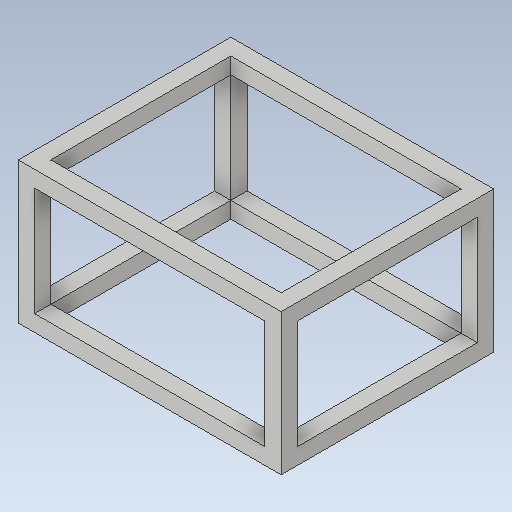
# Autodesk Inventor part: Turning motor housing
Saved by Autodesk Inventor 2020 (Build 240168000, 168)
## iProperties
Created: 2020-10-15
Part Number: Turning motor housing
Material: Generic
Document SubType Name: Modeling
Designer: nabee
Density: 1 g/cm^3
Appearance: Default
Author: nabee
Autodesk Inventor part; units mm, degrees
ref_plane "YZ Plane" through (0, 0, 0) normal (1, 0, 0) x (0, 1, 0)
ref_plane "XZ Plane" through (0, 0, 0) normal (0, 1, 0) x (-1, 0, 0)
ref_plane "XY Plane" through (0, 0, 0) normal (0, 0, 1) x (1, 0, 0)
sketch "Sketch1" plane through (0, 0, 0) normal (0, 0, 1) x (1, 0, 0)
  line L0 (0, 0) -> (322.448, 0)
  line L1 (322.448, 0) -> (322.448, 173.35)
  line L2 (322.448, 173.35) -> (0, 173.35)
  line L3 (0, 173.35) -> (0, 0)
  dimension "d0" = 322.448
  dimension "d1" = 173.35
  constraints: 8 end point, 2 parallel, 1 horizontal, 1 perpendicular
  measures "d0" distance of L2.end L1.end
  measures "d1" distance of L2.end L0.start
extrude "Extrusion1" add sketch "Sketch1" along normal blind 260.725
sketch "Sketch2" plane through (0, 0, 260.725) normal (0, 0, 1) x (1, 0, 0)
  line L0 (20, 153.35) -> (302.448, 153.35)
  line L1 (302.448, 153.35) -> (302.448, 20)
  line L2 (302.448, 20) -> (20, 20)
  line L3 (20, 20) -> (20, 153.35)
  line L4 (322.448, 173.35) -> (0, 173.35) projected
  line L5 (0, 173.35) -> (0, 0) projected
  line L6 (0, 0) -> (322.448, 0) projected
  line L7 (322.448, 0) -> (322.448, 173.35) projected
  dimension "d4" = 20
  dimension "d5" = 20
  dimension "d6" = 20
  dimension "d7" = 20
  constraints: 8 end point, 2 parallel, 1 horizontal, 1 perpendicular
  measures "d4" distance between parallel lines of L4 L0
  measures "d5" distance between parallel lines of L5 L3
  measures "d6" distance between parallel lines of L6 L2
  measures "d7" distance between parallel lines of L7 L1
extrude "Extrusion2" cut sketch "Sketch2" against normal blind 900 contours L0 L1 L2 L3
sketch "Sketch3" plane through (322.448, 0, 0) normal (1, 0, 0) x (0, 0, -1)
  line L0 (-240.725, 153.35) -> (-20, 153.35)
  line L1 (-20, 153.35) -> (-20, 20)
  line L2 (-20, 20) -> (-240.725, 20)
  line L3 (-240.725, 20) -> (-240.725, 153.35)
  line L4 (0, 173.35) -> (-260.725, 173.35) projected
  line L5 (-260.725, 0) -> (-260.725, 173.35) projected
  line L6 (0, 0) -> (-260.725, 0) projected
  line L7 (0, 0) -> (0, 173.35) projected
  dimension "d10" = 20
  dimension "d11" = 20
  dimension "d12" = 20
  dimension "d13" = 20
  constraints: 8 end point, 2 parallel, 1 horizontal, 1 perpendicular
  measures "d10" distance between parallel lines of L4 L0
  measures "d11" distance between parallel lines of L5 L3
  measures "d12" distance between parallel lines of L6 L2
  measures "d13" distance between parallel lines of L7 L1
extrude "Extrusion3" cut sketch "Sketch3" against normal blind 900 contours L0 L1 L2 L3
sketch "Sketch4" plane through (0, 173.35, 0) normal (0, 1, 0) x (1, 0, 0)
  line L0 (20, -20) -> (302.448, -20)
  line L1 (302.448, -20) -> (302.448, -240.725)
  line L2 (302.448, -240.725) -> (20, -240.725)
  line L3 (20, -240.725) -> (20, -20)
  line L4 (322.448, 0) -> (0, 0) projected
  line L5 (0, 0) -> (0, -260.725) projected
  line L6 (322.448, 0) -> (322.448, -260.725) projected
  line L7 (322.448, -260.725) -> (0, -260.725) projected
  dimension "d16" = 20
  dimension "d17" = 20
  dimension "d18" = 20
  dimension "d19" = 20
  constraints: 8 end point, 2 parallel, 1 horizontal, 1 perpendicular
  measures "d16" distance between parallel lines of L4 L0
  measures "d17" distance between parallel lines of L5 L3
  measures "d18" distance between parallel lines of L6 L1
  measures "d19" distance between parallel lines of L7 L2
extrude "Extrusion4" cut sketch "Sketch4" against normal blind 900 contours L0 L1 L2 L3
body "Solid1"
